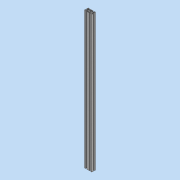
# Autodesk Inventor part: Profil dolny posuwu osi Y
Saved by Autodesk Inventor 2018 (Build 220112000, 112)
## iProperties
Created: 2019-01-25
Part Number: Profil dolny posuwu osi Y
Material: Ogólny
Document SubType Name: Modeling
Designer: Dawid
Density: 1 g/cm^3
Appearance: Aluminium odlewane
Author: Dawid
Autodesk Inventor part; units mm, degrees
ref_plane "YZ Plane" through (0, 0, 0) normal (1, 0, 0) x (0, 1, 0)
ref_plane "XZ Plane" through (0, 0, 0) normal (0, 1, 0) x (-1, 0, 0)
ref_plane "XY Plane" through (0, 0, 0) normal (0, 0, 1) x (1, 0, 0)
sketch "Szkic1" plane through (0, 0, 0) normal (0, 0, 1) x (1, 0, 0)
  circle A0 centre (-10, 9.9979) radius 2.1
  line L0 (-14.9613, 3.9784) -> (-13.0228, 5.9005)
  line L1 (-18.0066, 4.5634) -> (-18.0066, 6.2992)
  line L2 (-18.0066, 13.7008) -> (-18.0066, 15.4396)
  line L3 (-14.9613, 3.9784) -> (-15.433, 3.5107)
  line L4 (-13.7036, 2.0034) -> (-15.4393, 2.0108)
  line L5 (-13.5697, 14.6303) -> (-15.4393, 16.5)
  line L6 (-13.5697, 14.6303) -> (-13.0393, 14.1)
  line L7 (-14.641, 13.5721) -> (-14.1103, 13.0421)
  line L8 (-13.7022, 18.0033) -> (-15.4393, 18.0033)
  line L9 (-14.641, 13.5721) -> (-16.5118, 15.4406)
  line L10 (-15.4393, 18.0033) -> (-15.4393, 16.5)
  line L11 (-18.0066, 15.4396) -> (-16.5118, 15.4406)
  line L12 (-18.0066, 4.5634) -> (-16.5066, 4.5634)
  line L13 (-15.4393, 2.0108) -> (-15.433, 3.5107)
  line L14 (-6.4303, 14.6303) -> (-6.9607, 14.1)
  line L15 (-5.3697, 13.5744) -> (-5.9, 13.044)
  line L16 (-5.8834, 4.8399) -> (-6.9441, 5.9005)
  line L17 (0, 2.0047) -> (-0.9393, 2.0047)
  line L18 (0, 18.0047) -> (-0.9393, 18.0047)
  line L19 (-6.4303, 14.6303) -> (-4.5607, 16.5)
  line L20 (-3.0607, 18.0047) -> (-3.0607, 15.8834)
  line L21 (-3.0607, 18.0047) -> (-0.9393, 18.0047)
  line L22 (-5.3697, 13.5744) -> (-3.0607, 15.8834)
  line L23 (-3.0607, 2.0047) -> (-3.0607, 4.126)
  line L24 (-5.8834, 4.8399) -> (-4.5441, 3.5005)
  line L25 (-3.0607, 2.0047) -> (-0.9393, 2.0047)
  line L26 (-14.1088, 10.5027) -> (-14.1103, 13.0421)
  line L27 (-10.5, 14.1) -> (-13.0393, 14.1)
  line L28 (-9.5, 14.1) -> (-6.9607, 14.1)
  line L29 (-5.9, 10.5047) -> (-5.9, 13.044)
  line L30 (-5.9, 9.5047) -> (-5.9, 6.9653)
  line L31 (-9.4834, 5.9005) -> (-6.9441, 5.9005)
  line L32 (-10.4834, 5.9005) -> (-13.0228, 5.9005)
  arc A1 (-10.5, 14.1) -> (-9.5, 14.1) centre (-10, 14.6) ccw
  arc A2 (-14.1066, 9.5043) -> (-14.1088, 10.5027) centre (-14.6085, 10.0024) ccw
  arc A3 (-9.4834, 5.9005) -> (-10.4834, 5.9005) centre (-9.9834, 5.4005) ccw
  arc A4 (-5.9, 10.5047) -> (-5.9, 9.5047) centre (-5.4, 10.0047) ccw
  line L33 (10.4902, 5.8988) -> (13.0296, 5.903)
  arc A5 (5.9005, 9.5022) -> (5.9009, 10.5022) centre (5.4007, 10.0024) ccw
  circle A6 centre (10.0007, 9.9979) radius 2.1
  line L34 (5.9009, 10.5022) -> (5.902, 13.0415)
  line L35 (9.5024, 14.096) -> (6.9631, 14.097)
  line L36 (6.433, 14.6276) -> (6.9631, 14.097)
  arc A7 (14.1196, 10.4757) -> (14.1201, 9.5001) centre (14.6318, 9.9882) ccw
  arc A8 (9.5024, 14.096) -> (10.5024, 14.0955) centre (10.0026, 14.5957) ccw
  line L37 (14.1196, 10.4757) -> (14.1074, 13.015)
  line L38 (10.5024, 14.0955) -> (13.0418, 14.0945)
  line L39 (14.6352, 13.5478) -> (14.1074, 13.015)
  line L40 (13.5723, 14.6246) -> (13.0418, 14.0945)
  line L41 (14.9631, 3.9759) -> (13.0296, 5.903)
  line L42 (15.4994, 6.8934) -> (15.1709, 6.8935) construction
  line L43 (14.9631, 3.9759) -> (15.4335, 3.507)
  line L44 (13.7003, 2.0034) -> (15.436, 2.007)
  line L45 (15.436, 2.007) -> (15.4335, 3.507)
  line L46 (18.0049, 4.5347) -> (16.505, 4.5441)
  arc A9 (10.4902, 5.8988) -> (9.4902, 5.8971) centre (9.991, 5.398) ccw
  line L47 (9.4902, 5.8971) -> (6.9509, 5.8929)
  line L48 (5.3719, 13.5721) -> (5.902, 13.0415)
  line L49 (5.3719, 13.5721) -> (3.0638, 15.8821)
  line L50 (6.433, 14.6276) -> (4.5641, 16.4981)
  line L51 (0, 18.0047) -> (0.9434, 18.0043)
  line L52 (3.0648, 18.0034) -> (0.9434, 18.0043)
  line L53 (3.0648, 18.0034) -> (3.0638, 15.8821)
  line L54 (4.5648, 18.004) -> (4.5641, 16.4981)
  line L55 (5.9005, 9.5022) -> (5.8994, 6.9628)
  line L56 (5.892, 4.8305) -> (6.9509, 5.8929)
  line L57 (5.892, 4.8305) -> (4.5549, 3.4889)
  line L58 (18.0049, 13.6979) -> (17.9959, 15.4336)
  line L59 (13.5723, 14.6246) -> (15.4516, 16.5103)
  line L60 (13.7076, 18.0033) -> (15.4433, 18.0136)
  line L61 (14.6352, 13.5478) -> (16.4959, 15.4264)
  line L62 (15.4433, 18.0136) -> (15.4516, 16.5103)
  line L63 (17.9959, 15.4336) -> (16.4959, 15.4264)
  line L64 (3.0579, 2.0034) -> (3.0588, 4.1247)
  line L65 (3.0579, 2.0034) -> (0.9366, 2.0043)
  line L66 (0, 2.0047) -> (0.9366, 2.0043)
  line L67 (-4.5607, 16.5) -> (-4.5607, 18.0033)
  line L68 (-6.2912, 18.0033) -> (-4.5607, 18.0033)
  line L69 (6.3005, 18.0033) -> (4.5648, 18.004)
  line L70 (-14.1066, 9.5043) -> (-14.1066, 6.9634)
  line L71 (14.1201, 9.5001) -> (14.1201, 6.9592)
  line L72 (3.0588, 4.1247) -> (5.8994, 6.9628)
  line L73 (-5.9, 6.9653) -> (-3.0607, 4.126)
  line L74 (-4.5441, 2.0034) -> (-6.2916, 2.0034)
  line L75 (-4.5441, 3.5005) -> (-4.5441, 2.0034)
  line L76 (4.5549, 2.0034) -> (6.3661, 2.0034)
  line L77 (6.5461, 1.5766) -> (6.5038, 1.5343)
  line L78 (4.5549, 3.4889) -> (4.5549, 2.0034)
  line L79 (-20, 18.0132) -> (-20, 18.0033)
  line L80 (-15.2296, 20.026) -> (-19.5, 20.026)
  line L81 (19.5, 20.026) -> (15.2462, 20.026)
  line L82 (4.7627, 20.026) -> (-4.7651, 20.026)
  line L83 (20, 0.526) -> (20, 4.7886)
  line L84 (20, 15.1962) -> (20, 19.526)
  line L85 (15.1853, 0.026) -> (19.5, 0.026)
  line L86 (-19.5, 0.026) -> (-15.1868, 0.026)
  line L87 (-4.8035, 0.026) -> (4.8919, 0.026)
  line L88 (-20, 19.526) -> (-20, 15.2036)
  line L89 (-20, 4.7964) -> (-20, 0.526)
  line L90 (-16.5066, 4.5634) -> (-14.1066, 6.9634)
  line L91 (16.505, 4.5441) -> (14.1201, 6.9592)
  line L92 (-8.9462, 9.9979) -> (-8.9325, 9.9979)
  arc A10 (-19.5, 20.026) -> (-20, 19.526) centre (-19.5, 19.526) ccw
  arc A11 (20, 19.526) -> (19.5, 20.026) centre (19.5, 19.526) ccw
  arc A12 (19.5, 0.026) -> (20, 0.526) centre (19.5, 0.526) ccw
  arc A13 (-20, 0.526) -> (-19.5, 0.026) centre (-19.5, 0.526) ccw
  line L93 (-12.6, 20.026) -> (-12.6, 18.0033)
  line L94 (-7.4, 20.026) -> (-7.4, 18.0033)
  line L95 (-4.7651, 20.026) -> (-7.4, 20.026)
  line L96 (-12.6, 20.026) -> (-15.2296, 20.026)
  line L97 (-13.7022, 18.0033) -> (-12.6, 18.0033)
  line L98 (-7.4, 18.0033) -> (-6.2912, 18.0033)
  line L99 (-20, 12.6) -> (-18.0066, 12.6)
  line L100 (-18.0066, 12.6) -> (-18.0066, 13.7008)
  line L101 (-20, 7.4) -> (-18.0066, 7.4)
  line L102 (-18.0066, 7.4) -> (-18.0066, 6.2992)
  line L103 (-20, 15.2036) -> (-20, 12.6)
  line L104 (-20, 7.4) -> (-20, 4.7964)
  line L105 (-7.4, 0.026) -> (-7.4, 2.0034)
  line L106 (-7.4, 2.0034) -> (-6.2916, 2.0034)
  line L107 (-12.6, 0.026) -> (-12.6, 2.0034)
  line L108 (-12.6, 2.0034) -> (-13.7036, 2.0034)
  line L109 (-15.1868, 0.026) -> (-12.6, 0.026)
  line L110 (-7.4, 0.026) -> (-4.8035, 0.026)
  line L111 (7.4007, 20.026) -> (4.7627, 20.026)
  line L112 (15.2462, 20.026) -> (12.6007, 20.026)
  line L113 (12.6007, 20.026) -> (12.6007, 18.0033)
  line L114 (12.6007, 18.0033) -> (13.7076, 18.0033)
  line L115 (7.4007, 20.026) -> (7.4007, 18.0033)
  line L116 (7.4007, 18.0033) -> (6.3005, 18.0033)
  line L117 (20, 7.3979) -> (20, 4.7886)
  line L118 (20, 12.5979) -> (20, 15.1962)
  line L119 (20, 12.5979) -> (18.0049, 12.5979)
  line L120 (18.0049, 12.5979) -> (18.0049, 13.6979)
  line L121 (20, 7.4) -> (20, 7.3979)
  line L122 (20, 7.3979) -> (18.0049, 7.3979)
  line L123 (18.0049, 7.3979) -> (18.0049, 4.5347)
  line L124 (10.0007, 9.9979) -> (19.9726, 9.9979) construction
  line L125 (12.6007, 0.026) -> (15.1853, 0.026)
  line L126 (4.8919, 0.026) -> (7.4007, 0.026)
  line L127 (12.6007, 0.026) -> (12.6007, 2.0034)
  line L128 (12.6007, 2.0034) -> (13.7003, 2.0034)
  line L129 (7.4007, 0.026) -> (7.4007, 2.0034)
  line L130 (7.4007, 2.0034) -> (6.3661, 2.0034)
  constraints: 262 end point, 24 perpendicular, 24 point on circle, 14 centre point, 13 horizontal, 13 parallel, 12 point on line, 9 vertical, 8 tangent, 5 collinear, 3 equal radius
extrude "Wyciągnięcie proste1" add sketch "Szkic1" along normal blind 720
